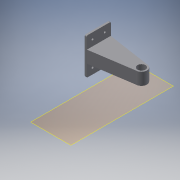
# Autodesk Inventor part: soporte
Saved by Autodesk Inventor 2016 (Build 200138000, 138)
## iProperties
Created: 2020-03-18
Part Number: soporte
Material: Genérico
Document SubType Name: Modeling
Designer: Andres Gomez
Density: 1 g/cm^3
Appearance: Valor por defecto
Author: Andres Gomez
Autodesk Inventor part; units mm, degrees
ref_plane "YZ Plane" through (0, 0, 0) normal (1, 0, 0) x (0, 1, 0)
ref_plane "XZ Plane" through (0, 0, 0) normal (0, 1, 0) x (-1, 0, 0)
ref_plane "XY Plane" through (0, 0, 0) normal (0, 0, 1) x (1, 0, 0)
ref_plane "Plano de trabajo1" through (0, 0, 0) normal (0, 0, 1) x (1, 0, 0)
sketch "Boceto1" plane through (0, 0, 0) normal (0, 0, 1) x (1, 0, 0)
  circle A0 centre (-9.9048, 81.1277) radius 6.5
  line L0 (-79.9048, 100.693) -> (-79.9048, 87.6277)
  line L1 (-79.9048, 74.6277) -> (-79.9048, 61.5627)
  line L2 (-79.9048, 87.6277) -> (-79.9048, 74.6277)
  circle A1 centre (-9.9048, 81.1277) radius 9
  line L3 (-79.9048, 100.693) -> (-9.9048, 90.1277)
  line L4 (-79.9048, 61.5627) -> (-9.9048, 72.1277)
  point P0 (0, 0)
  dimension "d0" = 13
  dimension "d2" = 13.065
  dimension "d3" = 18
  constraints: 10 end point, 2 centre point, 2 point on circle, 1 coincident, 1 collinear, 1 point on line, 1 vertical
  measures "d0" diameter of A0
  measures "d2" distance of L1.start L1.end
  measures "d3" diameter of A1
extrude "Extrusión1" add sketch "Boceto1" along normal blind 20
sketch "Boceto2" plane through (-79.9048, 61.5627, 0) normal (-1, 0, 0) x (0, 0, 1)
  line L0 (0, 39.1303) -> (0, 0) projected
  line L1 (20, 39.1303) -> (20, 0) projected
  line L2 (0, 39.1303) -> (20, 0)
  line L3 (20, 39.1303) -> (0, 0)
  line L4 (40, -0.4348) -> (-20, -0.4348)
  line L5 (-20, -0.4348) -> (-20, 39.5652)
  line L6 (-20, 39.5652) -> (40, 39.5652)
  line L7 (40, 39.5652) -> (40, -0.4348)
  line L8 (40, -0.4348) -> (-20, 39.5652) construction
  line L9 (-20, -0.4348) -> (40, 39.5652) construction
  point P0 (0, -61.5627)
  point P1 (10, 19.5652)
  dimension "d6" = 60
  dimension "d7" = 40
  constraints: 16 end point, 3 midpoint, 2 parallel, 1 horizontal, 1 perpendicular
  measures "d6" distance of L5.end L6.end
  measures "d7" distance of L4.end L5.end
extrude "Extrusión2" add sketch "Boceto2" along normal blind 3 contours L2 L3 L0 | L3 L1 L2 | L4 L5 L6 L7
fillet "Empalme1" radius 2 4 edges at (-81.4048, 101.1278, -20) (-81.4048, 101.1278, 40) (-81.4048, 61.1278, -20) (-81.4048, 61.1278, 40)
sketch "Boceto4" plane through (-82.9048, 61.5627, 0) normal (-1, 0, 0) x (0, 0, 1)
  line L0 (-10.1021, 39.6035) -> (-10.1021, 29.6035)
  line L1 (-10.1021, 29.6035) -> (-20.1021, 29.6035)
  circle A0 centre (-10.1021, 29.6035) radius 1.7
  line L2 (-10.1021, 29.6035) -> (-10.1021, -0.4348)
  line L3 (38, -0.4348) -> (-18, -0.4348) projected
  line L4 (-10.1021, -0.4348) -> (-10.1021, 9.5652)
  line L5 (-10.1021, 9.5652) -> (40.1083, 9.5652)
  line L6 (40.1083, 9.5652) -> (30.1083, 9.5652)
  line L7 (30.1083, 9.5652) -> (30.1083, 39.6035)
  line L8 (30.1083, 39.6035) -> (30.1083, 29.6035)
  circle A1 centre (-10.1021, 9.5652) radius 1.7
  circle A2 centre (30.1083, 9.5652) radius 1.7
  circle A3 centre (30.1083, 29.6035) radius 1.7
  point P0 (0, -61.5627)
  dimension "d11" = 10
  dimension "d12" = 10
  dimension "d13" = 3.4
  dimension "d14" = 10
  dimension "d15" = 10
  dimension "d16" = 10
  dimension "d17" = 3.4
  dimension "d18" = 3.4
  dimension "d19" = 3.4
  constraints: 16 end point, 4 centre point, 4 coincident, 4 point on line, 3 perpendicular, 2 vertical
  measures "d11" distance of L0.start L0.end
  measures "d12" distance of L0.end L1.end
  measures "d13" diameter of A0
  measures "d14" distance of L2.end L4.end
  measures "d15" distance of L5.end L6.end
  measures "d16" distance of L7.end L8.end
  measures "d17" diameter of A1
  measures "d18" diameter of A2
  measures "d19" diameter of A3
extrude "Extrusión3" cut sketch "Boceto4" against normal blind 3
sketch "Boceto5" plane through (0, 0, 20) normal (0, 0, 1) x (1, 0, 0)
  circle A0 centre (-9.8912, 81.0888) radius 7
  point P0 (0, 0)
  dimension "d22" = 14
  constraints: 1 centre point
  measures "d22" diameter of A0
extrude "Extrusión4" add sketch "Boceto5" against normal blind 5
sketch "Boceto6" plane through (0, 0, 0) normal (0, 0, -1) x (-1, 0, 0)
  circle A0 centre (-4.1803, 81.1277) radius 12.4106
  point P0 (0, 0)
  constraints: 1 centre point
extrude "Extrusión5" cut sketch "Boceto6" against normal blind 20
fillet "Empalme2" radius 0.5 5 edges at (-6.83, 75.4009, 7.5) (-6.83, 86.8544, 7.5) (-5.4544, 88.9504, 10) (-5.4544, 73.305, 10) (-8.2303, 81.1277, 20)
